Autodesk Fusion 360 part; units mm, degrees
(part 2 of 2)
sketch "Sketch15" plane through (0, -246.6728, 0) normal (0, -1, 0) x (1, 0, 0)
  line L0 (153.25, 0.5) -> (153.25, 9.1)
  line L1 (153.25, 9.1) -> (149, 9.1)
  line L2 (149, 9.1) -> (149, 6)
  line L3 (149, 6) -> (143, 6)
  line L4 (143, 6) -> (143, 9.1)
  line L5 (143, 9.1) -> (138, 9.1)
  line L6 (138, 9.1) -> (138, 6)
  line L7 (138, 6) -> (88, 6)
  line L8 (88, 6) -> (88, 9.1)
  line L9 (88, 9.1) -> (83, 9.1)
  line L10 (83, 9.1) -> (83, 6)
  line L11 (83, 6) -> (77, 6)
  line L12 (77, 6) -> (77, 9.1)
  line L13 (77, 9.1) -> (72, 9.1)
  line L14 (72, 9.1) -> (72, 0.5)
  line L15 (72, 0.5) -> (84.9436, 0.5)
  line L16 (84.9436, 0.5) -> (84.9436, -2)
  line L17 (84.9436, -2) -> (139.5734, -2)
  line L18 (139.5734, -2) -> (139.5734, 0.5)
  line L19 (139.5734, 0.5) -> (153.25, 0.5)
  circle A0 centre (92, 6) radius 2
  circle A1 centre (134, 6) radius 2
  line L20 (154, 0.5) -> (154, 9.1)
  circle A2 centre (113, 6) radius 2
  line L21 (92, 6) -> (113, 6) construction
  line L22 (113, 6) -> (134, 6) construction
  line L23 (92, 6) -> (113, 5.5) construction
  line L24 (113, 5.5) -> (134, 6) construction
  line L25 (113, 6) -> (113, 5.5) construction
  dimension "d303" = 4
  dimension "d304" = 8
  dimension "d305" = 20
  dimension "d306" = 4
  dimension "d307" = 20
  dimension "d310" = 4
  constraint coincident L7 A1.centre
  constraint coincident L7 A2.centre
  constraint coincident A0.centre L21.start
  constraint coincident A2.centre L21.end
  constraint coincident A1.centre L22.end
  constraint vertical L25
  constraint equal L23 L24
  measures "d303" diameter of A0
  measures "d304" distance of L17 A0.centre
  measures "d305" distance of L14 A0.centre
  measures "d306" diameter of A1
  measures "d307" distance of A1.centre L20
  measures "d310" diameter of A2
extrude "Extrude18" add sketch "Sketch15" along normal blind 6 contours L7 A1 | L7 A0 picked at (134.3298, 4.8074) picked at (91.9576, 5.2358) bodies 1
sketch "Sketch16" plane through (0, 0, 6) normal (0, 0, 1) x (-1, 0, 0)
  line L0 (-83, 246.6728) -> (-83, 241.6728)
  line L1 (-83, 241.6728) -> (-88, 241.6728)
  line L2 (-88, 241.6728) -> (-88, 246.6728)
  line L3 (-88, 246.6728) -> (-90, 246.6728)
  line L4 (-90, 246.6728) -> (-90, 252.6728)
  line L5 (-90, 252.6728) -> (-94, 252.6728)
  line L6 (-94, 252.6728) -> (-94, 246.6728)
  line L7 (-94, 246.6728) -> (-132, 246.6728)
  line L8 (-132, 246.6728) -> (-132, 252.6728)
  line L9 (-132, 252.6728) -> (-136, 252.6728)
  line L10 (-136, 252.6728) -> (-136, 246.6728)
  line L11 (-136, 246.6728) -> (-138, 246.6728)
  line L12 (-138, 246.6728) -> (-138, 241.6728)
  line L13 (-138, 241.6728) -> (-100.5171, 241.6728)
  arc A0 (-72, 236.7154) -> (-100.5171, 241.6728) centre (-100.5171, 157.1728) ccw
  line L14 (-72, 236.7154) -> (-72, 241.6728)
  line L15 (-72, 241.6728) -> (-77, 241.6728)
  line L16 (-77, 241.6728) -> (-77, 246.6728)
  line L17 (-77, 246.6728) -> (-83, 246.6728)
  line L18 (-90, 252.6728) -> (-94, 252.6728)
  line L19 (-94, 252.6728) -> (-94, 250.6728)
  line L20 (-94, 250.6728) -> (-90, 250.6728)
  line L21 (-90, 250.6728) -> (-90, 252.6728)
  line L22 (-111, 252.6728) -> (-115, 252.6728)
  line L23 (-115, 252.6728) -> (-115, 250.6728)
  line L24 (-115, 250.6728) -> (-111, 250.6728)
  line L25 (-111, 250.6728) -> (-111, 252.6728)
  line L26 (-132, 252.6728) -> (-136, 252.6728)
  line L27 (-136, 252.6728) -> (-136, 250.6728)
  line L28 (-136, 250.6728) -> (-132, 250.6728)
  line L29 (-132, 250.6728) -> (-132, 252.6728)
  dimension "d311" = 2
  dimension "d312" = 4
  dimension "d313" = 2
  dimension "d314" = 4
  dimension "d315" = 2
  dimension "d318" = 4
  constraint horizontal L18
  constraint vertical L19
  constraint horizontal L20
  constraint vertical L21
  constraint coincident L4.end L5.start
  constraint horizontal L22
  constraint vertical L23
  constraint horizontal L24
  constraint vertical L25
  constraint horizontal L26
  constraint vertical L27
  constraint horizontal L28
  constraint vertical L29
  constraint coincident L8.end L9.start
  measures "d311" distance of L4.end L20.end
  measures "d312" distance of L22.start L22.end
  measures "d313" distance of L22.start L24.end
  measures "d314" distance of L8.end L9.end
  measures "d315" distance of L8.end L28.end
  measures "d318" distance of L4.end L5.end
extrude "Extrude19" add sketch "Sketch16" against normal up to surface (8 mm away) contours L4 L5 L6 L18 L19 L20 L21 | L8 L9 L10 L26 L27 L28 L29 bodies 1
sketch "Sketch6" plane through (0, 0, 11.5) normal (0, 0, 1) x (-1, 0, 0) in component "Component"
  line L0 (-143.5, 226.6728) -> (-143.5, 247.1728)
  line L1 (-143.5, 247.1728) -> (-148.5, 247.1728)
  line L2 (-148.5, 247.1728) -> (-148.5, 226.6728)
  line L3 (-148.5, 226.6728) -> (-154, 226.6728)
  line L4 (-154, 226.6728) -> (-154, 188)
  line L5 (-154, 188) -> (-118, 188)
  line L6 (-118, 188) -> (-118, 178)
  line L7 (-118, 178) -> (-108, 178)
  line L8 (-108, 178) -> (-108, 188)
  line L9 (-108, 188) -> (-72, 188)
  line L10 (-72, 188) -> (-72, 226.6728)
  line L11 (-72, 226.6728) -> (-77.5, 226.6728)
  line L12 (-77.5, 226.6728) -> (-77.5, 247.1728)
  line L13 (-77.5, 247.1728) -> (-82.5, 247.1728)
  line L14 (-82.5, 247.1728) -> (-82.5, 226.6728)
  line L15 (-82.5, 226.6728) -> (-143.5, 226.6728)
  circle A0 centre (-148.5195, 217.7511) radius 1.6
  circle A1 centre (-112.5195, 217.7511) radius 1.6
  circle A2 centre (-76.5195, 217.7511) radius 1.6
  circle A3 centre (-132.5195, 217.7511) radius 1.6
  dimension "d319" = 3.2
  dimension "d323" = 72
  dimension "d324" = 0
  dimension "d327" = 16
  dimension "d328" = 0
  dimension "d329" = 5.4805
  measures "d319" diameter of A0
  measures "d329" distance of L4 A0.centre
extrude "Extrude9" cut sketch "Sketch6" against normal up to surface (3 mm away) contours A0 | A1 | A2 | A3 bodies 13 in component "Component"
extrude "Extrude20" add 1 faces at (88, -244.2151, 6.4349) along direction (1, 0, 0) blind 15 on bodies 1 bodies 1
extrude "Extrude21" add 1 faces at (138, -244.2151, 6.4349) along direction (-1, 0, 0) blind 15 on bodies 1 bodies 1
component "Component" placed x (1, 0, 0) y (0, 1, 0) z (0, 0, 1) at (0, 0, 0)
equation "d155 = d154"
equation "d287 = 8.517 mm - 4 mm"
